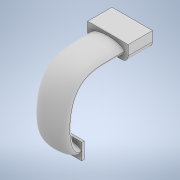
# Autodesk Inventor part: Verbindung_Motor_Servo
Saved by Autodesk Inventor 2021 (Build 250183000, 183)
## iProperties
Created: 2021-01-04
Part Number: Verbindung_Motor_Servo
Material: Generisch
Document SubType Name: Modeling
Designer: Ctroi
Density: 1 g/cm^3
Appearance: Vorgabe
Mass: 91.5133 g
Surface Area: 197.408 cm^2
Volume: 91.5133 cm^3
Author: Ctroi
Autodesk Inventor part; units mm, degrees
ref_plane "YZ Plane" through (0, 0, 0) normal (1, 0, 0) x (0, 1, 0)
ref_plane "XZ Plane" through (0, 0, 0) normal (0, 1, 0) x (-1, 0, 0)
ref_plane "XY Plane" through (0, 0, 0) normal (0, 0, 1) x (1, 0, 0)
sketch "Skizze1" plane through (0, 0, 0) normal (0, 1, 0) x (-1, 0, 0)
  line L0 (25, -15) -> (-25, -15)
  line L1 (-25, -15) -> (-25, 15)
  line L2 (-25, 15) -> (25, 15)
  line L3 (25, 15) -> (25, -15)
  line L4 (35, 0) -> (-35, 0) projected
  line L5 (0, -21) -> (0, 21) projected
  point P0 (0, 0)
  dimension "d0" = 50
  dimension "d1" = 30
  constraints: 8 end point, 2 parallel, 1 horizontal, 1 perpendicular, 2 other
  measures "d0" distance of L1.end L2.end
  measures "d1" distance of L0.end L1.end
extrude "Extrusion1" add sketch "Skizze1" along normal blind 3
ref_plane "Arbeitsebene1" through (-25, 0, 65) normal (0, 0, 1) x (1, 0, 0)
sketch "Skizze3" plane through (-25, 0, 65) normal (0, 0, 1) x (1, 0, 0)
  line L0 (4.25, -60) -> (45.75, -60)
  line L1 (45.75, -60) -> (45.75, -80)
  line L2 (45.75, -80) -> (4.25, -80)
  line L3 (4.25, -80) -> (4.25, -60)
  line L4 (25, 0) -> (25, -85.9898)
  line L5 (50, 0) -> (0, 0) projected
  dimension "d8" = 41.5
  dimension "d9" = 20
  dimension "d16" = 60
  constraints: 10 end point, 2 parallel, 1 horizontal, 1 perpendicular, 1 vertical, 1 other
  measures "d8" distance of L1.end L2.end
  measures "d9" distance of L0.end L1.end
  measures "d16" distance between parallel lines of L5 L0
extrude "Extrusion3" add sketch "Skizze3" along normal blind 3
sketch "Skizze7" plane through (0, 3, 0) normal (0, 1, 0) x (1, 0, 0)
  point P0 (0, 0)
extrude "Extrusion6" add sketch "Skizze1" along normal blind 20
sketch "Skizze8" plane through (-25, 0, 15) normal (0, 0, 1) x (1, 0, 0)
  ellipse E0 centre (25, 10) end of major axis (45, 10) minor radius 7
  line L0 (50, 0) -> (50, 20) projected
  line L1 (50, 10) -> (0, 10)
  line L2 (0, 0) -> (0, 20) projected
  line L3 (50, 0) -> (0, 0) projected
  line L4 (0, 10) -> (50, 10)
  point P0 (25, 0)
  dimension "d25" = 20
  dimension "d26" = 7
  dimension "d38" = 10
  constraints: 4 end point, 4 midpoint, 1 centre point, 1 perpendicular
  measures "d25" diameter of E0
  measures "d38" distance from line of L3 E0.centre
sketch "Skizze9" plane through (0, 0, 0) normal (1, 0, 0) x (0, 1, 0)
  line L0 (0, 15) -> (20, 15) projected
  line L1 (-80, 68) -> (-60, 68) projected
  line L2 (-60, 68) -> (-80, 68) projected
  spline S0 degree 4 poles (10, 15) (9.5883, 70.4749) (18.2812, 84.2128) (-72.49, 92.1756) (-70, 68) knots 0 0 0 0 0 1 1 1 1 1
  line L3 (10.1796, -9.2022) -> (9.8204, 39.2022) construction
  arc A0 (10.5195, 34.3212) -> (10.8062, -4.3113) centre (291.7825, 17.0911) ccw construction
  point P0 (0, 0)
  point P1 (-0.3605, 69.8283)
  point P2 (-45.2501, 81.8124)
  constraints: 4 midpoint, 2 end point, 1 centre point, 1 point on circle, 6 other
fillet "Rundung1" radius 8 2 edges at (-25, 0, 0) (25, 0, 0)
sweep "Sweeping4" add profiles "Skizze8" path "Skizze9" path curves S0 contours L1 E0 | E0 L1
